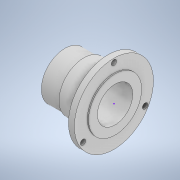
# Autodesk Inventor part: parte eixo
Saved by Autodesk Inventor 2022.1 (Build 261234020, 234B)
## iProperties
Created: 2023-08-25
Part Number: parte eixo
Material: Generic
Document SubType Name: Modeling
Designer: SENAI
Density: 1 g/cm^3
Appearance: Default
Author: SENAI
Autodesk Inventor part; units mm, degrees
ref_plane "YZ Plane" through (0, 0, 0) normal (1, 0, 0) x (0, 1, 0)
ref_plane "XZ Plane" through (0, 0, 0) normal (0, 1, 0) x (-1, 0, 0)
ref_plane "XY Plane" through (0, 0, 0) normal (0, 0, 1) x (1, 0, 0)
sketch "Sketch1" plane through (0, 0, 0) normal (0, 0, 1) x (1, 0, 0)
  line L0 (0, 0) -> (0, 40)
  line L1 (0, 40) -> (32, 40)
  line L2 (32, 40) -> (32, 42)
  line L3 (73, 67) -> (73, 47)
  line L4 (73, 47) -> (32, 42)
  line L5 (83, 67) -> (83, 45)
  line L6 (83, 45) -> (85, 45)
  line L7 (83, 67) -> (73, 67)
  line L8 (85, 0) -> (0, 0)
  line L9 (85, 45) -> (85, 0)
  dimension "d1" = 40
  dimension "d2" = 32
  dimension "d4" = 10
  dimension "d5" = 2
  dimension "d6" = 20
  dimension "d9" = 22
  dimension "d10" = 2
  dimension "d11" = 85
  constraints: 20 end point, 5 vertical, 2 horizontal, 2 perpendicular
  measures "d1" distance of L0.start L0.end
  measures "d2" distance of L0.end L1.end
  measures "d4" distance of L5.start L3.start
  measures "d5" distance of L1.end L2.end
  measures "d6" distance of L3.start L3.end
  measures "d9" distance of L5.start L5.end
  measures "d10" distance of L5.end L6.end
  measures "d11" distance of L8.start L0.start
revolve "Revolution1" add sketch "Sketch1" angle 360 about axis through (85, 0, 0) along (-1, 0, 0)
sketch "Sketch2" plane through (85, 0, 0) normal (1, 0, 0) x (0, 0, -1)
  circle A0 centre (0, 0) radius 30
  dimension "d13" = 60
  constraints: 1 centre point, 1 coincident
  measures "d13" diameter of A0
extrude "Extrusion1" cut sketch "Sketch2" against normal blind 86
sketch "Sketch3" plane through (85, 0, 0) normal (1, 0, 0) x (0, 0, -1)
  circle A0 centre (0, 60.5) radius 4.5
  circle A1 centre (52.8551, -29.5948) radius 4.5
  circle A2 centre (-52.3945, -30.25) radius 4.5
  circle A3 centre (0, 0) radius 47 projected
  circle A4 centre (0, 0) radius 67 projected
  line L0 (58.0237, -33.5) -> (56.2917, -32.5)
  dimension "d17" = 9
  dimension "d16" = 9
  dimension "d18" = 9
  dimension "d23" = 2
  constraints: 2 centre point, 2 end point, 5 other
  measures "d16" diameter of A0
  measures "d18" diameter of A2
  measures "d23" distance of L0.start L0.end
sketch "Sketch4" plane through (83, 0, 0) normal (1, 0, 0) x (0, 0, -1)
  point P0 (0, 0)
extrude "Extrusion2" cut sketch "Sketch3" against normal blind 86 contours A0 | A1 | A2
body "Solid1"
